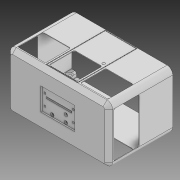
# Autodesk Inventor part: Cablecar_frame
Saved by Autodesk Inventor 2020 (Build 240168000, 168)
## iProperties
Created: 2021-02-03
Part Number: Cablecar_frame
Material: Generic
Document SubType Name: Modeling
Designer: DDeGo
Density: 1 g/cm^3
Appearance: Default
Author: DDeGo
Autodesk Inventor part; units mm, degrees
ref_plane "YZ Plane" through (0, 0, 0) normal (1, 0, 0) x (0, 1, 0)
sketch "Sketch1" plane through (0, 0, 0) normal (0, 0, 1) x (1, 0, 0)
  line L0 (-90, -50) -> (90, -50)
  line L1 (90, -50) -> (90, 50)
  line L2 (90, 50) -> (-90, 50)
  line L3 (-90, 50) -> (-90, -50)
  line L4 (-90, -50) -> (90, 50) construction
  line L5 (90, -50) -> (-90, 50) construction
  point P0 (0, 0)
  dimension "d0" = 180
  dimension "d1" = 100
  constraints: 12 end point, 2 midpoint, 2 parallel, 1 horizontal, 1 perpendicular
  measures "d0" distance of L1.end L2.end
  measures "d1" distance of L0.end L1.end
extrude "Extrusion1" add sketch "Sketch1" along normal blind 120
fillet "Fillet1" radius 10 4 edges at (90, -50, 60) (-90, -50, 60) (90, 50, 60) (-90, 50, 60)
chamfer "Chamfer1" distance 7 angle 45 16 edges at (0, -50, 0) (87.0711, -47.0711, 0) (90, 0, 0) (87.0711, 47.0711, 0) (0, 50, 0) (-87.0711, 47.0711, 0) (-90, 0, 0) (-87.0711, -47.0711, 0) (0, -50, 120) (87.0711, -47.0711, 120) (90, 0, 120) (87.0711, 47.0711, 120) (0, 50, 120) (-87.0711, 47.0711, 120) (-90, 0, 120) (-87.0711, -47.0711, 120)
ref_plane "Work Plane1" through (-45, -50, 113) normal (0, 0, 1) x (1, 0, 0)
sketch "Sketch2" plane through (0, 0, 0) normal (0, 0, -1) x (-1, 0, 0)
  line L0 (-80, -50) -> (80, -50) construction
  arc A0 (80, -50) -> (90, -40) centre (80, -40) ccw construction
  line L1 (90, -40) -> (90, 40) construction
  line L2 (-90, 40) -> (-90, -40) construction
  arc A1 (-90, -40) -> (-80, -50) centre (-80, -40) ccw construction
  arc A2 (-80, 50) -> (-90, 40) centre (-80, 40) ccw construction
  line L3 (80, 50) -> (-80, 50) construction
  arc A3 (90, 40) -> (80, 50) centre (80, 40) ccw construction
  line L4 (80, -49) -> (-80, -49)
  arc A4 (-89, -40) -> (-80, -49) centre (-80, -40) ccw
  line L5 (-89, -40) -> (-89, 40)
  arc A5 (-80, 49) -> (-89, 40) centre (-80, 40) ccw
  line L6 (-80, 49) -> (80, 49)
  arc A6 (89, 40) -> (80, 49) centre (80, 40) ccw
  line L7 (89, 40) -> (89, -40)
  arc A7 (80, -49) -> (89, -40) centre (80, -40) ccw
  point P0 (0, 0)
  dimension "d8" = 1
  constraints: 8 end point, 8 point on circle, 4 centre point, 7 other
  measures "d8" distance between parallel lines of L0 L4
extrude "Extrusion2" cut sketch "Sketch2" against normal up to surface (113 mm away)
sketch "Sketch3" plane through (-80, -50, 113) normal (0, -1, 0) x (1, 0, 0)
  line L0 (160, 0) -> (0, 0) construction
  line L1 (160, -106) -> (0, -106) construction
  line L2 (0, 0) -> (53.3333, 0) construction
  line L3 (53.3333, -106) -> (0, -106) construction
  line L4 (53.3333, -106) -> (106.6667, -106) construction
  line L5 (106.6667, 0) -> (53.3333, 0) construction
  line L6 (106.6667, 0) -> (160, 0) construction
  line L7 (160, -106) -> (106.6667, -106) construction
  line L8 (3, -2) -> (46.3333, -2)
  line L9 (49.3333, -5) -> (49.3333, -44)
  line L10 (46.3333, -47) -> (3, -47)
  line L11 (0, -44) -> (0, -5)
  line L12 (58.3333, -2) -> (101.6667, -2)
  line L13 (104.6667, -5) -> (104.6667, -44)
  line L14 (101.6667, -47) -> (58.3333, -47)
  line L15 (55.3333, -44) -> (55.3333, -5)
  line L16 (113.6667, -2) -> (157, -2)
  line L17 (160, -5) -> (160, -44)
  line L18 (157, -47) -> (113.6667, -47)
  line L19 (110.6667, -44) -> (110.6667, -5)
  arc A0 (0, -44) -> (3, -47) centre (3, -44) ccw
  arc A1 (46.3333, -47) -> (49.3333, -44) centre (46.3333, -44) ccw
  arc A2 (55.3333, -44) -> (58.3333, -47) centre (58.3333, -44) ccw
  arc A3 (101.6667, -47) -> (104.6667, -44) centre (101.6667, -44) ccw
  arc A4 (110.6667, -44) -> (113.6667, -47) centre (113.6667, -44) ccw
  arc A5 (157, -47) -> (160, -44) centre (157, -44) ccw
  arc A6 (160, -5) -> (157, -2) centre (157, -5) ccw
  arc A7 (113.6667, -2) -> (110.6667, -5) centre (113.6667, -5) ccw
  arc A8 (104.6667, -5) -> (101.6667, -2) centre (101.6667, -5) ccw
  arc A9 (58.3333, -2) -> (55.3333, -5) centre (58.3333, -5) ccw
  arc A10 (49.3333, -5) -> (46.3333, -2) centre (46.3333, -5) ccw
  arc A11 (3, -2) -> (0, -5) centre (3, -5) ccw
  line L20 (0, -106) -> (0, 0) construction
  line L21 (160, 0) -> (160, -106) construction
  point P0 (80, -113)
  point P1 (0, -2)
  point P2 (49.3333, -47)
  point P3 (49.3333, -2)
  point P4 (0, -47)
  point P5 (55.3333, -2)
  point P6 (104.6667, -47)
  point P7 (104.6667, -2)
  point P8 (55.3333, -47)
  point P9 (110.6667, -2)
  point P10 (160, -47)
  point P11 (160, -2)
  point P12 (110.6667, -47)
  dimension "d11" = 2
  dimension "d16" = 6
  dimension "d17" = 45
  dimension "d18" = 6
  dimension "d21" = 3
  constraints: 36 end point, 28 point on line, 24 point on circle, 24 tangent, 12 centre point, 11 equal radius, 9 collinear, 9 parallel, 6 horizontal, 3 perpendicular
  measures "d11" distance between parallel lines of L2 L8
  measures "d16" distance between parallel lines of L15 L9
  measures "d17" distance of point (104.667, -2) point (104.667, -47)
  measures "d18" distance between parallel lines of L13 L19
  measures "d21" radius of A0
extrude "Extrusion3" cut sketch "Sketch3" against normal blind 3
sketch "Sketch4" plane through (-80, -50, 113) normal (0, -1, 0) x (1, 0, 0)
  line L0 (52.8333, -1.5) -> (107.1667, -1.5)
  line L1 (107.1667, -1.5) -> (107.1667, -104)
  line L2 (107.1667, -104) -> (52.8333, -104)
  line L3 (52.8333, -104) -> (52.8333, -1.5)
  line L4 (58.3333, -2) -> (101.6667, -2) construction
  line L5 (49.3333, -5) -> (49.3333, -44) construction
  line L6 (55.3333, -44) -> (55.3333, -5) construction
  line L7 (51.8333, -0.5) -> (108.1667, -0.5)
  line L8 (108.1667, -0.5) -> (108.1667, -105)
  line L9 (108.1667, -105) -> (51.8333, -105)
  line L10 (51.8333, -105) -> (51.8333, -0.5)
  line L11 (104.6667, -5) -> (104.6667, -44) construction
  line L12 (160, -106) -> (0, -106) construction
  circle A0 centre (101.6667, -52.5588) radius 2.3217
  point P0 (80, -113)
  dimension "d22" = 0.5
  dimension "d23" = 6
  dimension "d24" = 2.5
  dimension "d25" = 1
  dimension "d26" = 2.5
  dimension "d27" = 1
  constraints: 16 end point, 4 parallel, 2 perpendicular, 1 centre point, 1 horizontal, 3 other
  measures "d22" distance between parallel lines of L4 L0
  measures "d23" distance between parallel lines of L5 L6
  measures "d24" distance between parallel lines of L6 L3
  measures "d25" distance between parallel lines of L3 L10
  measures "d26" distance between parallel lines of L1 L11
  measures "d27" distance between parallel lines of L12 L9
extrude "Extrusion4" cut sketch "Sketch4" against normal blind 0.2
sketch "Sketch5" plane through (90, -40, 113) normal (1, 0, 0) x (0, 0, -1)
  line L0 (5, 0) -> (44, 0)
  line L1 (47, 3) -> (47, 77)
  line L2 (44, 80) -> (5, 80)
  line L3 (2, 77) -> (2, 3)
  line L4 (106, 0) -> (0, 0) construction
  line L5 (0, 80) -> (106, 80) construction
  line L6 (0, 0) -> (0, 80) construction
  arc A0 (2, 3) -> (5, 0) centre (5, 3) ccw
  arc A1 (5, 80) -> (2, 77) centre (5, 77) ccw
  arc A2 (47, 77) -> (44, 80) centre (44, 77) ccw
  arc A3 (44, 0) -> (47, 3) centre (44, 3) ccw
  point P0 (113, 40)
  point P1 (47, -10)
  dimension "d30" = 2
  dimension "d31" = 3
  constraints: 8 end point, 8 point on circle, 8 tangent, 4 centre point, 3 equal radius, 2 collinear, 2 parallel, 1 horizontal, 1 perpendicular, 1 point on line
  measures "d30" distance between parallel lines of L6 L3
  measures "d31" radius of A0
extrude "Extrusion5" cut sketch "Sketch5" against normal through all
mirror "Mirror1" about plane through (0, 0, 0) normal (0, 1, 0) of "Extrusion3", "Extrusion4"
sketch "Sketch6" plane through (0, 0, 120) normal (0, 0, 1) x (1, 0, 0)
  line L0 (30, -20) -> (-30, -20)
  line L1 (-30, -20) -> (-30, 20)
  line L2 (-30, 20) -> (30, 20)
  line L3 (30, 20) -> (30, -20)
  line L4 (30, -20) -> (-30, 20) construction
  line L5 (-30, -20) -> (30, 20) construction
  point P0 (0, 0)
  dimension "d34" = 40
  dimension "d35" = 60
  constraints: 12 end point, 2 midpoint, 2 parallel, 1 horizontal, 1 perpendicular
  measures "d34" distance of L0.end L1.end
  measures "d35" distance of L1.end L2.end
extrude "Extrusion6" cut sketch "Sketch6" against normal blind 2.6
sketch "Sketch7" plane through (0, 0, 117.4) normal (0, 0, 1) x (1, 0, 0)
  line L0 (25, -10) -> (-25, -10) construction
  line L1 (-25, -10) -> (-25, 10) construction
  line L2 (-25, 10) -> (25, 10) construction
  line L3 (25, 10) -> (25, -10) construction
  line L4 (25, -10) -> (-25, 10) construction
  line L5 (-25, -10) -> (25, 10) construction
  circle A0 centre (-25, 10) radius 1.75
  circle A1 centre (-25, -10) radius 1.75
  circle A2 centre (25, -10) radius 1.75
  circle A3 centre (25, 10) radius 1.75
  point P0 (0, 0)
  dimension "d38" = 3.5
  dimension "d39" = 20
  dimension "d40" = 50
  constraints: 12 end point, 4 centre point, 4 coincident, 3 equal radius, 2 midpoint, 2 parallel, 1 horizontal, 1 perpendicular
  measures "d38" diameter of A0
  measures "d39" distance of L0.end L1.end
  measures "d40" distance of L1.end L2.end
extrude "Extrusion7" cut sketch "Sketch7" against normal through all
sketch "Sketch8" plane through (0, 0, 117.4) normal (0, 0, 1) x (1, 0, 0)
  line L0 (0, 0) -> (0, 4.5) construction
  line L1 (-22.5, 6) -> (22.5, 6)
  line L2 (22.5, 6) -> (22.5, 3)
  line L3 (22.5, 3) -> (-22.5, 3)
  line L4 (-22.5, 3) -> (-22.5, 6)
  line L5 (-22.5, 6) -> (22.5, 3) construction
  line L6 (22.5, 6) -> (-22.5, 3) construction
  dimension "d43" = 4.5
  dimension "d44" = 3
  dimension "d45" = 45
  constraints: 14 end point, 2 midpoint, 2 parallel, 1 horizontal, 1 perpendicular, 1 vertical
  measures "d43" distance of L0.start L0.end
  measures "d44" distance of L3.end L1.start
  measures "d45" distance of L1.start L1.end
extrude "Extrusion8" cut sketch "Sketch8" against normal through all
sketch "Sketch9" plane through (80, 49, 113) normal (0, 0, -1) x (-1, 0, 0)
  line L0 (57.5, -43) -> (57.5, -46) projected
  line L1 (57.5, -44.5) -> (80, -44.5) construction
  line L2 (80, -44.5) -> (80, -59.5) construction
  line L3 (68, -65.5) -> (92, -65.5) construction
  line L4 (92, -65.5) -> (92, -53.5) construction
  line L5 (92, -53.5) -> (68, -53.5) construction
  line L6 (68, -53.5) -> (68, -65.5) construction
  line L7 (68, -65.5) -> (92, -53.5) construction
  line L8 (92, -65.5) -> (68, -53.5) construction
  circle A0 centre (68, -53.5) radius 1.65
  circle A1 centre (68, -65.5) radius 1.65
  circle A2 centre (92, -65.5) radius 1.65
  point P0 (80, -49)
  dimension "d48" = 12
  dimension "d49" = 24
  dimension "d50" = 3.3
  dimension "d51" = 15
  constraints: 16 end point, 3 centre point, 3 coincident, 3 midpoint, 2 equal radius, 2 horizontal, 2 parallel, 2 perpendicular, 1 point on line
  measures "d48" distance of L5.end L3.start
  measures "d49" distance of L4.end L5.end
  measures "d50" diameter of A0
  measures "d51" distance of L1.end L2.end
extrude "Extrusion9" cut sketch "Sketch9" against normal through all
sketch "Sketch11" plane through (0, 0, 117.4) normal (0, 0, 1) x (1, 0, 0)
  circle A0 centre (-12, -16.5) radius 1.65 projected
  circle A1 centre (-12, -16.5) radius 3
  circle A2 centre (12, -16.5) radius 1.65 projected
  circle A3 centre (12, -16.5) radius 3
  circle A4 centre (12, -4.5) radius 1.65 projected
  circle A5 centre (12, -4.5) radius 3
  point P0 (0, 0)
  dimension "d57" = 6
  constraints: 3 centre point, 3 coincident, 2 equal radius
  measures "d57" diameter of A1
extrude "Extrusion11" cut sketch "Sketch11" against normal blind 3 contours A0 | A1 | A2 | A3 | A4 | A5
ref_plane "Work Plane2" through (-62.5, -49, 6) normal (0, 0, -1) x (1, 0, 0)
sketch "Sketch12" plane through (-62.5, -49, 6) normal (0, 0, -1) x (1, 0, 0)
  circle A0 centre (74.5, -44.5) radius 1.65 construction
  circle A1 centre (74.5, -32.5) radius 1.65 construction
  circle A2 centre (50.5, -32.5) radius 1.65 construction
  line L0 (40, -55) -> (40, -52) construction
  line L1 (40, -52) -> (85, -52) construction
  line L2 (85, -52) -> (85, -55) construction
  line L3 (85, -55) -> (40, -55) construction
  circle A3 centre (87.5, -39) radius 1.75 construction
  circle A4 centre (37.5, -39) radius 1.75 construction
  circle A5 centre (37.5, -59) radius 1.75 construction
  circle A6 centre (87.5, -59) radius 1.75 construction
  line L4 (-26.5, -9) -> (-26.5, -89) construction
  arc A7 (-26.5, -89) -> (-17.5, -98) centre (-17.5, -89) ccw construction
  line L5 (-17.5, -98) -> (142.5, -98) construction
  arc A8 (142.5, -98) -> (151.5, -89) centre (142.5, -89) ccw construction
  line L6 (151.5, -89) -> (151.5, -9) construction
  arc A9 (151.5, -9) -> (142.5, 0) centre (142.5, -9) ccw construction
  line L7 (142.5, 0) -> (-17.5, 0) construction
  arc A10 (-17.5, 0) -> (-26.5, -9) centre (-17.5, -9) ccw construction
  arc A11 (-17.5, 0) -> (-26.5, -9) centre (-17.5, -9) ccw construction
  line L8 (-26.4497, -8.0503) -> (-21.4497, -8.0503)
  line L9 (-18.4497, -5.0503) -> (-18.4497, -0.0503)
  arc A12 (-18.4497, -0.0503) -> (-26.4497, -8.0503) centre (-17.5, -9) ccw
  arc A13 (-21.4497, -8.0503) -> (-18.4497, -5.0503) centre (-21.4497, -5.0503) ccw
  circle A14 centre (-21.4497, -5.0503) radius 1.5
  line L10 (62.5, 0) -> (62.5, -49) construction
  line L11 (62.5, -49) -> (-26.5, -49) construction
  line L12 (-26.5, -89) -> (-26.5, -9) projected
  line L13 (151.4497, -8.0503) -> (146.4497, -8.0503)
  line L14 (143.4497, -5.0503) -> (143.4497, -0.0503)
  arc A15 (151.4497, -8.0503) -> (143.4497, -0.0503) centre (142.5, -9) ccw
  arc A16 (143.4497, -5.0503) -> (146.4497, -8.0503) centre (146.4497, -5.0503) ccw
  circle A17 centre (146.4497, -5.0503) radius 1.5
  line L15 (142.5, -98) -> (-17.5, -98) construction
  line L16 (-26.4497, -89.9497) -> (-21.4497, -89.9497)
  line L17 (-18.4497, -92.9497) -> (-18.4497, -97.9497)
  arc A18 (-26.4497, -89.9497) -> (-18.4497, -97.9497) centre (-17.5, -89) ccw
  arc A19 (-18.4497, -92.9497) -> (-21.4497, -89.9497) centre (-21.4497, -92.9497) ccw
  circle A20 centre (-21.4497, -92.9497) radius 1.5
  line L18 (151.4497, -89.9497) -> (146.4497, -89.9497)
  arc A21 (146.4497, -89.9497) -> (143.4497, -92.9497) centre (146.4497, -92.9497) ccw
  circle A22 centre (146.4497, -92.9497) radius 1.5
  line L19 (143.4497, -92.9497) -> (143.4497, -97.9497)
  arc A23 (143.4497, -97.9497) -> (151.4497, -89.9497) centre (142.5, -89) ccw
  point P0 (-18.4497, -8.0503)
  point P1 (143.4497, -8.0503)
  point P2 (-18.4497, -89.9497)
  point P3 (62.5, -98)
  point P4 (143.4497, -89.9497)
  dimension "d60" = 8
  dimension "d61" = 3
  dimension "d62" = 3
  constraints: 25 symmetric about line, 22 end point, 18 point on circle, 12 centre point, 8 point on line, 4 coincident, 2 midpoint, 2 perpendicular, 2 tangent, 1 concentric, 1 horizontal, 1 vertical, 9 other
  measures "d60" distance of point (-18.45, -8.05) L9.end
  measures "d61" radius of A13
  measures "d62" diameter of A14
extrude "Extrusion12" add sketch "Sketch12" against normal blind 5 contours A12 L9 A13 L8 | A14 | L13 A16 L14 A15 | A17 | L16 A19 L17 A18 | A20 | A23 L19 A21 L18 | A22
chamfer "Chamfer2" distance 6.4 angle 45 4 edges at (-86.364, -46.364, 11) (-86.364, 46.364, 11) (86.364, -46.364, 11) (86.364, 46.364, 11)
sketch "Sketch13" plane through (-62.5, -49, 6) normal (0, 0, -1) x (-1, 0, 0)
  arc A0 (-143.4497, 5.0503) -> (-146.4497, 8.0503) centre (-146.4497, 5.0503) ccw projected
  circle A1 centre (-146.4497, 5.0503) radius 1.425
  arc A2 (-146.4497, 89.9497) -> (-143.4497, 92.9497) centre (-146.4497, 92.9497) ccw projected
  circle A3 centre (-146.4497, 92.9497) radius 1.425
  arc A4 (18.4497, 92.9497) -> (21.4497, 89.9497) centre (21.4497, 92.9497) ccw projected
  circle A5 centre (21.4497, 92.9497) radius 1.425
  arc A6 (21.4497, 8.0503) -> (18.4497, 5.0503) centre (21.4497, 5.0503) ccw projected
  circle A7 centre (21.4497, 5.0503) radius 1.425
  point P0 (-62.5, 49)
  dimension "d68" = 2.85
  constraints: 4 centre point, 4 coincident, 3 equal radius
  measures "d68" diameter of A1
extrude "Extrusion13" cut sketch "Sketch13" against normal blind 20
equation "\"d18\" = d16"
equation "\"d24\" = -0.5 * d25 + 0.5 * d23"
equation "\"d26\" = d24"
body "Solid1"
